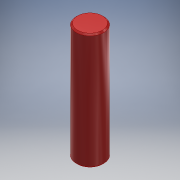
# Autodesk Inventor part: Perno forcella
Saved by Autodesk Inventor 2018 (Build 220112000, 112)
## iProperties
Created: 2020-06-12
Part Number: Perno forcella
Material: Acciaio inossidabile
Document SubType Name: Modeling
Designer: Francesco
Density: 8 g/cm^3
Appearance: Rosso
Author: Francesco
Autodesk Inventor part; units mm, degrees
ref_plane "YZ Plane" through (0, 0, 0) normal (1, 0, 0) x (0, 1, 0)
ref_plane "XZ Plane" through (0, 0, 0) normal (0, 1, 0) x (-1, 0, 0)
ref_plane "XY Plane" through (0, 0, 0) normal (0, 0, 1) x (1, 0, 0)
sketch "Schizzo1" plane through (0, 0, 0) normal (0, 0, 1) x (1, 0, 0)
  circle A0 centre (0, 0) radius 5
  dimension "d0" = 10
  constraints: 1 centre point, 1 coincident
  measures "d0" diameter of A0
extrude "Estrusione1" add sketch "Schizzo1" along normal mid plane 42
chamfer "Smusso1" distance 0.5 angle 45 2 edges at (-5, 0, 21) (-5, 0, -21)
